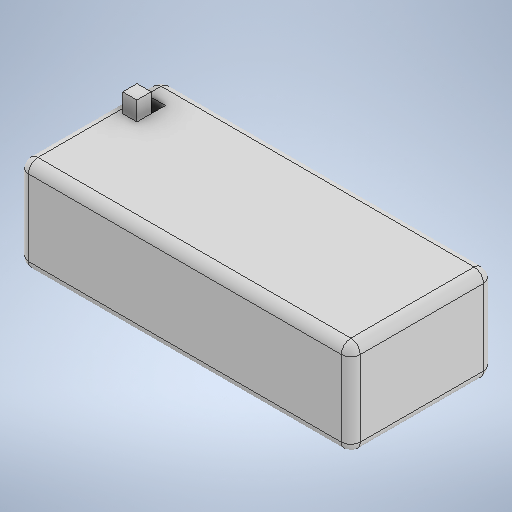
# Autodesk Inventor part: Part6
Saved by Autodesk Inventor 2025.2 (Build 292293000, 293)
## iProperties
Created: 2025-04-15
Part Number: Part6
Material: Generic
Document SubType Name: Sheet Metal
Designer: ziyuz
Density: 1 g/cm^3
Sheet Metal Rule: Default_mm
Appearance: Default
Author: ziyuz
Autodesk Inventor part; units mm, degrees
ref_plane "YZ Plane" through (0, 0, 0) normal (1, 0, 0) x (0, 1, 0)
ref_plane "XZ Plane" through (0, 0, 0) normal (0, 1, 0) x (-1, 0, 0)
ref_plane "XY Plane" through (0, 0, 0) normal (0, 0, 1) x (1, 0, 0)
sketch "Sketch1" plane through (0, 0, 0) normal (0, 1, 0) x (-1, 0, 0)
  line L0 (0, 0) -> (70, 0)
  line L1 (70, 0) -> (70, -30)
  line L2 (70, -30) -> (0, -30)
  line L3 (0, -30) -> (0, 0)
  dimension "d0" = 70
  dimension "d1" = 30
  constraints: 8 end point, 2 parallel, 1 horizontal, 1 perpendicular
  measures "d0" distance of L1.end L2.end
  measures "d1" distance of L0.end L1.end
extrude "Extrusion1" add sketch "Sketch1" along normal blind 20
fillet "Fillet1" radius 2 11 edges at (-70, 10, 0) (-70, 20, -15) (-35, 20, 0) (-70, 0, -15) (-35, 0, 0) (0, 10, 0) (0, 20, -15) (0, 0, -15) (0, 10, -30) (-35, 20, -30) (-35, 0, -30)
sketch "Sketch2" plane through (0, 20, 0) normal (0, 1, 0) x (1, 0, 0)
  line L0 (-67.0416, 18.9322) -> (-64.0416, 18.9322)
  line L1 (-64.0416, 18.9322) -> (-64.0416, 24.9322)
  line L2 (-64.0416, 24.9322) -> (-67.0416, 24.9322)
  line L3 (-67.0416, 24.9322) -> (-67.0416, 18.9322)
  point P0 (0, 0)
  dimension "d6" = 3
  dimension "d7" = 6
  constraints: 8 end point, 2 parallel, 1 horizontal, 1 perpendicular
  measures "d6" distance of L2.end L1.end
  measures "d7" distance of L1.end L0.end
fillet "Fillet2" radius 2 3 edges at (-69.4142, 19.4142, -29.4142) (-69.4142, 0.5858, -29.4142) (-70, 10, -30)
extrude "Extrusion2" cut sketch "Sketch2" against normal blind 4
sketch "Sketch3" plane through (0, 16, 0) normal (0, 1, 0) x (1, 0, 0)
  line L0 (-64.0416, 18.9322) -> (-67.0416, 18.9322) projected
  line L1 (-67.0416, 18.9322) -> (-67.0416, 24.9322) projected
  line L2 (-64.0416, 18.9322) -> (-67.0416, 18.9322)
  line L3 (-67.0416, 18.9322) -> (-67.0416, 21.9322)
  line L4 (-67.0416, 21.9322) -> (-64.0416, 21.9322)
  line L5 (-64.0416, 21.9322) -> (-64.0416, 18.9322)
  point P0 (0, 0)
  constraints: 8 end point, 2 parallel, 1 horizontal, 1 midpoint, 1 perpendicular
extrude "Extrusion3" add sketch "Sketch3" along normal blind 8
equation "\"BendRadius\" = Thickness"
equation "\"BendReliefWidth\" = Thickness"
equation "\"BendReliefDepth\" = 0.5 * Thickness"
equation "\"CornerReliefSize\" = 4 * Thickness"
equation "\"MinimumRemnant\" = 2 * Thickness"
equation "\"TransitionRadius\" = BendRadius"
equation "\"JacobiRadiusSize\" = BendRadius"
equation "\"GapSize\" = Thickness"
equation "\"Thickness\" = 0.5"
body "Solid1"
